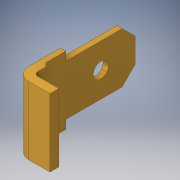
# Autodesk Inventor part: COM_Contact
Saved by Autodesk Inventor 2016 (Build 200138000, 138)
## iProperties
Created: 2016-05-07
Part Number: COM_Contact
Material: Brass, Soft Yellow
Document SubType Name: Modeling
Designer: agmle
Density: 8.47 g/cm^3
Appearance: Brass - Satin
Author: agmle
Autodesk Inventor part; units mm, degrees
ref_plane "YZ Plane" through (0, 0, 0) normal (1, 0, 0) x (0, 1, 0)
ref_plane "XZ Plane" through (0, 0, 0) normal (0, 1, 0) x (-1, 0, 0)
ref_plane "XY Plane" through (0, 0, 0) normal (0, 0, 1) x (1, 0, 0)
sketch "Sketch1" plane through (0, 0, 0) normal (0, 1, 0) x (-1, 0, 0)
  line L0 (0, 0) -> (0, -0.85)
  line L1 (0, -0.85) -> (2, -0.85)
  line L2 (2.4, -1.25) -> (2.4, -2)
  line L3 (2.4, -2) -> (2.75, -2.35)
  line L4 (2.75, -2.35) -> (2.75, -10.85)
  line L5 (2.75, -10.85) -> (3.25, -10.85)
  line L6 (3.25, -10.85) -> (3.25, -1.25)
  line L7 (2, 0) -> (0, 0)
  arc A0 (3.25, -1.25) -> (2, 0) centre (2, -1.25) ccw
  arc A1 (2.4, -1.25) -> (2, -0.85) centre (2, -1.25) ccw
  dimension "d1" = 0.85
  dimension "d2" = 0.5
  dimension "d3" = 3.25
  dimension "d4" = 10.85
  dimension "d5" = 1.25
  dimension "d6" = 135
  dimension "d7" = 8.5
  constraints: 16 end point, 5 perpendicular, 4 point on circle, 4 tangent, 2 centre point, 1 coincident, 1 parallel, 1 vertical
  measures "d1" distance of L0.start L0.end
  measures "d2" distance between parallel lines of L4 L6
  measures "d3" distance between parallel lines of L0 L6
  measures "d4" distance between parallel lines of L7 L5
  measures "d5" radius of A0
  measures "d6" angle of L4 L3
  measures "d7" distance from line of L5 L3.end
extrude "Extrusion1" add sketch "Sketch1" along normal blind 6.45
sketch "Sketch2" plane through (-3.25, 0, -10.85) normal (-1, 0, 0) x (0, 0, 1)
  line L0 (0, 0) -> (9.6, 0) projected
  line L1 (0, 0) -> (0, 6.45) projected
  line L2 (0, 6.45) -> (9.6, 6.45) projected
  line L3 (6.6, 0) -> (6.6, 0.825)
  line L4 (6.6, 0.825) -> (1.25, 0.825)
  line L5 (1.25, 0.825) -> (0, 2.075)
  line L6 (6.6, 6.45) -> (6.6, 5.625)
  line L7 (6.6, 5.625) -> (1.25, 5.625)
  line L8 (1.25, 5.625) -> (0, 4.375)
  line L9 (0, 0) -> (0, 6.45) projected
  line L10 (10.85, 0) -> (10.85, 6.45) projected
  circle A0 centre (3.27, 3.225) radius 0.72
  dimension "d10" = 135
  dimension "d11" = 4.8
  dimension "d12" = 1.25
  dimension "d13" = 4.25
  dimension "d14" = 1.44
  dimension "d15" = 3.27
  constraints: 12 end point, 6 point on line, 3 perpendicular, 2 equal length, 1 centre point, 1 vertical
  measures "d10" angle of L1 L5
  measures "d11" distance between parallel lines of L7 L4
  measures "d12" distance from line of L1 L4.end
  measures "d13" distance between parallel lines of L10 L3
  measures "d14" diameter of A0
  measures "d15" distance from line of L1 A0.centre
extrude "Extrusion2" cut sketch "Sketch2" against normal blind 6.45
body "Solid1"
